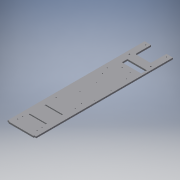
# Autodesk Inventor part: Control Board
Saved by Autodesk Inventor 2016 (Build 200138000, 138)
## iProperties
Created: 2017-09-15
Part Number: Control Board
Material: Generic
Document SubType Name: Modeling
Designer: Student
Density: 1 g/cm^3
Appearance: Default
Author: Student
Autodesk Inventor part; units mm, degrees
ref_plane "YZ Plane" through (0, 0, 0) normal (1, 0, 0) x (0, 1, 0)
ref_plane "XZ Plane" through (0, 0, 0) normal (0, 1, 0) x (-1, 0, 0)
ref_plane "XY Plane" through (0, 0, 0) normal (0, 0, 1) x (1, 0, 0)
sketch "Sketch1" plane through (0, 0, 0) normal (0, 1, 0) x (-1, 0, 0)
  line L0 (47.9603, 101.1149) -> (-52.1157, 101.1149)
  line L1 (-52.1157, 101.1149) -> (-52.1157, -254.4851)
  line L2 (-52.1157, -254.4851) -> (47.9603, -254.4851)
  line L3 (47.9603, -254.4851) -> (47.9603, 101.1149)
  point P0 (0, 0)
  dimension "d0" = 100.076
  dimension "d1" = 355.6
  constraints: 8 end point, 2 parallel, 1 horizontal, 1 perpendicular
  measures "d0" distance of L0.start L0.end
  measures "d1" distance of L2.end L0.start
extrude "Extrusion1" add sketch "Sketch1" along normal blind 5.4102
sketch "Sketch5" plane through (0, 5.4102, 0) normal (0, 1, 0) x (1, 0, 0)
  circle A0 centre (-34.7523, 244.8585) radius 1.5
  circle A1 centre (38.9077, 244.8585) radius 1.5
  line L0 (-34.7355, 243.3586) -> (38.8909, 243.3586)
  line L1 (52.1157, 254.4851) -> (-47.9603, 254.4851) projected
  point P0 (0, 0)
  point P1 (2.0777, 243.3586)
  point P2 (2.0777, 254.4851)
  dimension "d8" = 3
  dimension "d9" = 3
  dimension "d10" = 73.66
  dimension "d11" = 9.6266
  constraints: 2 end point, 2 midpoint, 1 horizontal, 1 vertical alignment, 6 other
  measures "d10" distance of point (38.908, 244.859) point (-34.752, 244.859)
  measures "d11" distance from line of L1 point (38.908, 244.859)
extrude "Extrusion3" cut sketch "Sketch5" against normal blind 25.4
sketch "Sketch6" plane through (0, 5.4102, 0) normal (0, 1, 0) x (1, 0, 0)
  line L0 (-47.9603, -101.1149) -> (52.1157, -101.1149) projected
  line L1 (-47.9603, -101.1149) -> (-41.6103, -101.1149)
  line L2 (-41.6103, -101.1149) -> (-41.6103, -98.3209)
  line L3 (-41.6103, -98.3209) -> (-47.9603, -98.3209)
  line L4 (-47.9603, -98.3209) -> (-47.9603, -101.1149)
  line L5 (52.1157, -101.1149) -> (45.7657, -101.1149)
  line L6 (45.7657, -101.1149) -> (45.7657, -98.3209)
  line L7 (45.7657, -98.3209) -> (52.1157, -98.3209)
  line L8 (52.1157, -98.3209) -> (52.1157, -101.1149)
  point P0 (0, 0)
  dimension "d14" = 2.794
  dimension "d15" = 6.35
  dimension "d16" = 6.35
  constraints: 16 end point, 4 parallel, 2 horizontal, 2 perpendicular, 1 point on line
  measures "d14" distance of L1.end L2.end
  measures "d15" distance of L2.end L3.end
  measures "d16" distance of L6.end L7.end
extrude "Extrusion4" cut sketch "Sketch6" against normal blind 25.4
sketch "Sketch7" plane through (45.7657, 5.4102, 98.3209) normal (0, 0, 1) x (1, 0, 0)
  circle A0 centre (3.175, -2.7051) radius 1.5
  line L0 (0, 0) -> (6.35, 0) projected
  line L1 (6.35, 0) -> (6.35, -5.4102) projected
  circle A1 centre (-90.551, -2.7051) radius 1.5
  line L2 (-93.726, 0) -> (-87.376, 0) projected
  line L3 (-93.726, -5.4102) -> (-93.726, 0) projected
  point P0 (-45.7657, -5.4102)
  point P1 (3.175, 0)
  point P2 (6.35, -2.7051)
  point P3 (-90.551, 0)
  point P4 (-93.726, -2.7051)
  dimension "d19" = 3
  dimension "d20" = 3
  constraints: 4 midpoint, 2 centre point, 2 horizontal alignment, 2 vertical alignment
  measures "d19" diameter of A0
  measures "d20" diameter of A1
extrude "Extrusion5" cut sketch "Sketch7" against normal blind 254
sketch "Sketch8" plane through (-41.6103, 0, 101.1149) normal (0, 0, 1) x (1, 0, 0)
  line L0 (0, 5.4102) -> (87.376, 5.4102) projected
  line L1 (0, 0) -> (87.376, 0) projected
  line L2 (0, 5.4102) -> (87.376, 5.4102)
  line L3 (87.376, 5.4102) -> (87.376, 0)
  line L4 (87.376, 0) -> (0, 0)
  line L5 (0, 0) -> (0, 5.4102)
  point P0 (41.6103, 0)
  constraints: 8 end point, 2 parallel, 1 horizontal, 1 perpendicular
extrude "Extrusion6" add sketch "Sketch8" along normal blind 54.5338
sketch "Sketch9" plane through (-47.9603, 5.4102, 98.3209) normal (0, 0, 1) x (1, 0, 0)
  line L0 (6.35, 0) -> (6.35, -5.4102) projected
  line L1 (0, 0) -> (6.35, 0)
  line L2 (6.35, 0) -> (6.35, -5.4102)
  line L3 (6.35, -5.4102) -> (0, -5.4102)
  line L4 (0, -5.4102) -> (0, 0)
  line L5 (100.076, 0) -> (100.076, -5.4102) projected
  line L6 (100.076, -5.4102) -> (93.726, -5.4102) projected
  line L7 (100.076, 0) -> (93.726, 0)
  line L8 (93.726, 0) -> (93.726, -5.4102)
  line L9 (93.726, -5.4102) -> (100.076, -5.4102)
  line L10 (100.076, -5.4102) -> (100.076, 0)
  circle A0 centre (96.901, -2.7051) radius 1.5
  circle A1 centre (3.175, -2.7051) radius 1.5
  point P0 (47.9603, -5.4102)
  constraints: 16 end point, 4 parallel, 2 centre point, 2 horizontal, 2 perpendicular
extrude "Extrusion7" add sketch "Sketch9" along normal blind 54.5338
sketch "Sketch10" plane through (0, 5.4102, 0) normal (0, 1, 0) x (1, 0, 0)
  line L0 (-37.6261, -131.8997) -> (38.5739, -131.8997) construction
  line L1 (-37.6261, -106.4997) -> (38.5739, -106.4997) construction
  line L2 (-47.9603, 254.4851) -> (-47.9603, -152.8547) construction
  line L3 (52.1157, -152.8547) -> (52.1157, 254.4851) construction
  line L4 (45.7657, -155.6487) -> (-41.6103, -155.6487) construction
  line L5 (-37.6261, -114.1197) -> (-12.2261, -114.1197) construction
  line L6 (-12.2261, -114.1197) -> (-12.2261, -124.2797) construction
  line L7 (-12.2261, -124.2797) -> (-37.6261, -124.2797) construction
  line L8 (-37.6261, -131.8997) -> (-37.6261, -124.2797) construction
  line L9 (-37.6261, -114.1197) -> (-37.6261, -106.4997) construction
  line L10 (38.5739, -114.1197) -> (13.1739, -114.1197) construction
  line L11 (13.1739, -114.1197) -> (13.1739, -124.2797) construction
  line L12 (13.1739, -124.2797) -> (38.5739, -124.2797) construction
  line L13 (38.5739, -131.8997) -> (38.5739, -124.2797) construction
  line L14 (38.5739, -114.1197) -> (38.5739, -106.4997) construction
  circle A0 centre (34.7639, -110.3097) radius 1.5
  circle A1 centre (34.7639, -128.0897) radius 1.5
  circle A2 centre (-33.816, -127.9782) radius 1.5
  circle A3 centre (-33.816, -110.1982) radius 1.5
  point P0 (0, 0)
  point P1 (38.5739, -110.3097)
  dimension "d27" = 76.2
  dimension "d28" = 25.4
  dimension "d31" = 23.749
  dimension "d32" = 7.62
  dimension "d33" = 7.62
  dimension "d34" = 25.4
  dimension "d35" = 25.4
  dimension "d36" = 68.58
  dimension "d37" = 17.78
  dimension "d38" = 17.78
  dimension "d39" = 68.58
  dimension "d40" = 3
  dimension "d41" = 3
  dimension "d42" = 3
  dimension "d43" = 3
  dimension "d44" = 3.81
  dimension "d45" = 25.4
  dimension "d46" = 25.4
  dimension "d47" = 7.62
  dimension "d48" = 7.62
  dimension "d49" = 7.62
  dimension "d50" = 7.62
  dimension "d51" = 76.2
  dimension "d52" = 25.4
  dimension "d53" = 25.4
  dimension "d54" = 17.78
  constraints: 24 end point, 12 perpendicular, 4 centre point, 2 horizontal, 2 vertical, 2 vertical alignment, 1 horizontal alignment, 1 midpoint
  measures "d27" distance of L1.start L1.end
  measures "d28" distance of L0.start L1.start
  measures "d31" distance between parallel lines of L4 L0
  measures "d32" distance between parallel lines of L1 L5
  measures "d33" distance between parallel lines of L7 L0
  measures "d34" distance of L5.start L5.end
  measures "d35" distance of L10.start L10.end
  measures "d36" distance of A3.centre A0.centre
  measures "d37" distance of A1.centre A0.centre
  measures "d38" distance of A3.centre A2.centre
  measures "d39" distance of A1.centre A2.centre
  measures "d40" diameter of A3
  measures "d41" diameter of A2
  measures "d42" diameter of A0
  measures "d43" diameter of A1
  measures "d44" distance from line of L14 A0.centre
  measures "d45" distance of L11.end L12.end
  measures "d46" distance of L6.end L7.end
  measures "d47" distance of L5.start L1.start
  measures "d48" distance of L10.start L1.end
  measures "d49" distance of L0.end L12.end
  measures "d50" distance of L0.start L7.end
  measures "d51" distance of L0.start L0.end
  measures "d52" distance between parallel lines of L11 L6
  measures "d53" distance between parallel lines of L0 L1
  measures "d54" distance of A2.centre A3.centre
extrude "Extrusion8" cut sketch "Sketch10" against normal blind 54.5338
sketch "Sketch11" plane through (0, 5.4102, 0) normal (0, 1, 0) x (1, 0, 0)
  line L0 (-41.6103, -155.6487) -> (45.7657, -155.6487) construction
  line L1 (43.9115, -155.6487) -> (43.9115, -13.9421) construction
  line L2 (43.9115, -13.9421) -> (52.1157, -13.9421) construction
  line L3 (52.1157, -152.8547) -> (52.1157, 254.4851) construction
  circle A0 centre (43.9115, -13.9421) radius 1.0922
  circle A1 centre (-7.8029, -13.9421) radius 1.0922
  circle A2 centre (43.9115, 43.9953) radius 1.0928
  circle A3 centre (-7.8029, 43.9953) radius 1.0922
  point P0 (0, 0)
  dimension "d57" = 141.7066
  dimension "d58" = 8.2042
  dimension "d59" = 2.1844
  dimension "d60" = 2.1844
  dimension "d62" = 51.7144
  dimension "d63" = 57.9374
  dimension "d64" = 57.9374
  constraints: 4 centre point, 4 end point, 2 point on line, 1 coincident, 1 perpendicular, 1 vertical
  measures "d57" distance of L1.start L1.end
  measures "d58" distance of L1.end L2.end
  measures "d59" diameter of A0
  measures "d60" diameter of A1
  measures "d62" distance of L1.end A1.centre
  measures "d63" distance of L1.end A2.centre
  measures "d64" distance of A3.centre A1.centre
extrude "Extrusion9" cut sketch "Sketch11" against normal blind 54.5338
sketch "Sketch12" plane through (0, 5.4102, 0) normal (0, 1, 0) x (1, 0, 0)
  circle A0 centre (43.4543, 73.8403) radius 1.5367
  line L0 (52.1157, -152.8547) -> (52.1157, 254.4851) projected
  line L1 (52.1157, -152.8547) -> (45.7657, -152.8547) projected
  line L2 (46.0959, 58.6257) -> (46.0959, 133.7589) construction
  line L3 (46.0959, 58.6257) -> (-7.3203, 58.6257) construction
  line L4 (46.0959, 133.7589) -> (44.0639, 133.7589) construction
  line L5 (44.0639, 133.7589) -> (44.0639, 136.7053) construction
  line L6 (44.0639, 136.7053) -> (6.6751, 136.7053) construction
  line L7 (6.6751, 136.7053) -> (6.6751, 133.7589) construction
  line L8 (6.6751, 133.7589) -> (-7.2949, 133.7589) construction
  line L9 (-7.3203, 58.6257) -> (-7.2949, 133.7589) construction
  circle A1 centre (38.5521, 134.0637) radius 1.5367
  circle A2 centre (10.6629, 134.0637) radius 1.5367
  point P0 (0, 0)
  dimension "d67" = 3.0734
  dimension "d68" = 8.6614
  dimension "d69" = 226.695
  dimension "d89" = 15.2146
  dimension "d90" = 2.6416
  dimension "d91" = 75.1332
  dimension "d92" = 53.4162
  dimension "d93" = 2.032
  dimension "d94" = 2.9464
  dimension "d95" = 37.3888
  dimension "d96" = 13.97
  dimension "d97" = 75.1332
  dimension "d98" = 3.0734
  dimension "d99" = 2.6416
  dimension "d100" = 3.0734
  dimension "d101" = 2.6416
  dimension "d102" = 27.8892
  dimension "d103" = 7.5438
  dimension "d104" = 60.4226
  constraints: 16 end point, 3 centre point, 3 horizontal, 3 vertical, 1 perpendicular
  measures "d67" diameter of A0
  measures "d68" distance from line of L0 A0.centre
  measures "d69" distance from line of A0.centre L1
  measures "d89" distance from line of L3 A0.centre
  measures "d90" distance from line of L2 A0.centre
  measures "d91" distance of L2.start L2.end
  measures "d92" distance of L2.start L3.end
  measures "d93" distance of L2.end L4.end
  measures "d94" distance of L4.end L5.end
  measures "d95" distance of L5.end L6.end
  measures "d96" distance of L7.end L8.end
  measures "d97" distance of L3.end L8.end
  measures "d98" diameter of A1
  measures "d99" distance from line of L6 A1.centre
  measures "d100" diameter of A2
  measures "d101" distance from line of L6 A2.centre
  measures "d102" distance of A1.centre A2.centre
  measures "d103" distance from line of L2 A1.centre
  measures "d104" distance of A1.centre A0.centre
extrude "Extrusion10" cut sketch "Sketch12" against normal blind 25.4
sketch "Sketch13" plane through (0, 5.4102, 0) normal (0, 1, 0) x (1, 0, 0)
  line L0 (44.9886, 149.6605) -> (-23.5191, 149.6605)
  line L1 (-23.5191, 149.6605) -> (-23.5191, 169.3907)
  line L2 (-23.5191, 169.3907) -> (44.9886, 169.3907)
  line L3 (44.9886, 169.3907) -> (44.9886, 149.6605)
  point P0 (0, 0)
  constraints: 8 end point, 2 parallel, 1 horizontal, 1 perpendicular
extrude "Extrusion11" cut sketch "Sketch13" against normal blind 25.4
sketch "Sketch14" plane through (0, 5.4102, 0) normal (0, 1, 0) x (1, 0, 0)
  line L0 (-39.2837, 182.0907) -> (45.1561, 182.0907) construction
  line L1 (45.1561, 182.0907) -> (45.1561, 192.9873) construction
  line L2 (45.1561, 192.9873) -> (-39.2837, 192.9873) construction
  line L3 (-39.2837, 192.9873) -> (-39.2837, 182.0907) construction
  line L4 (-23.5191, 169.3907) -> (44.9886, 169.3907) construction
  circle A0 centre (40.7951, 187.539) radius 2.2274
  circle A1 centre (-34.9227, 187.539) radius 2.2274
  line L5 (-47.9603, 254.4851) -> (-47.9603, -152.8547) construction
  line L6 (52.1157, -152.8547) -> (52.1157, 254.4851) construction
  point P0 (0, 0)
  dimension "d107" = 84.4398
  dimension "d108" = 10.8966
  dimension "d109" = 12.7
  dimension "d110" = 2.1336
  dimension "d111" = 2.1336
  dimension "d114" = 6.9596
  constraints: 8 end point, 3 perpendicular, 2 centre point, 1 horizontal
  measures "d107" distance of L1.end L2.end
  measures "d108" distance of L2.end L0.start
  measures "d109" distance between parallel lines of L4 L0
  measures "d110" distance edge to line of A0 L1
  measures "d111" distance edge to line of A1 L3
  measures "d114" distance between parallel lines of L6 L1
extrude "Extrusion12" cut sketch "Sketch14" against normal blind 25.4
sketch "Sketch15" plane through (0, 5.4102, 0) normal (0, 1, 0) x (1, 0, 0)
  circle A0 centre (30.5257, -47.4955) radius 1.5
  line L0 (-47.9603, 254.4851) -> (-47.9603, -152.8547) projected
  line L1 (-41.6103, -152.8547) -> (-47.9603, -152.8547) projected
  line L2 (52.1157, -152.8547) -> (52.1157, 254.4851) projected
  circle A1 centre (-24.0589, 81.4603) radius 1.5
  point P0 (0, 0)
  dimension "d117" = 3
  dimension "d119" = 105.3592
  dimension "d120" = 21.59
  dimension "d121" = 3
  dimension "d122" = 23.9014
  dimension "d123" = 234.315
  constraints: 2 centre point
  measures "d117" diameter of A0
  measures "d119" distance from line of L1 A0.centre
  measures "d120" distance from line of L2 A0.centre
  measures "d121" diameter of A1
  measures "d122" distance from line of L0 A1.centre
  measures "d123" distance from line of L1 A1.centre
extrude "Extrusion13" cut sketch "Sketch15" against normal blind 25.4
sketch "Sketch16" plane through (0, 0, 0) normal (0, -1, 0) x (1, 0, 0)
  line L0 (38.0609, 76.6965) -> (-35.2689, 76.6965)
  line L1 (-35.2689, 76.6965) -> (-35.2689, -110.1035)
  line L2 (-35.2689, -110.1035) -> (38.0609, -110.1035)
  line L3 (38.0609, -110.1035) -> (38.0609, 76.6965)
  circle A0 centre (35.0609, 73.6965) radius 1.5
  circle A1 centre (-32.2689, 73.6965) radius 1.5
  circle A2 centre (-32.2689, -107.1035) radius 1.5
  circle A3 centre (35.0609, -107.1035) radius 1.5
  point P0 (0, 0)
  dimension "d128" = 186.8
  dimension "d129" = 73.3298
  dimension "d130" = 3
  dimension "d131" = 3
  dimension "d132" = 3
  dimension "d133" = 3
  dimension "d134" = 3
  dimension "d135" = 3
  dimension "d136" = 3
  dimension "d137" = 3
  dimension "d138" = 3
  dimension "d139" = 3
  dimension "d140" = 3
  dimension "d141" = 3
  constraints: 8 end point, 4 centre point, 2 parallel, 1 horizontal, 1 perpendicular
  measures "d128" distance of L2.end L0.start
  measures "d129" distance of L1.end L2.end
  measures "d130" diameter of A0
  measures "d131" distance from line of L3 A0.centre
  measures "d132" distance from line of L0 A0.centre
  measures "d133" distance from line of L1 A1.centre
  measures "d134" distance from line of L0 A1.centre
  measures "d135" diameter of A1
  measures "d136" diameter of A2
  measures "d137" distance from line of L2 A2.centre
  measures "d138" distance from line of L1 A2.centre
  measures "d139" diameter of A3
  measures "d140" distance from line of L2 A3.centre
  measures "d141" distance from line of L3 A3.centre
extrude "Extrusion14" cut sketch "Sketch16" against normal blind 25.4 contours A0 | A1 | A2 | A3
sketch "Sketch17" plane through (-41.6103, 0, 155.6487) normal (0, 0, 1) x (1, 0, 0)
  line L0 (0, 5.4102) -> (0, 0) projected
  line L1 (0, 0) -> (87.376, 0) projected
  line L2 (0, 5.4102) -> (87.376, 5.4102)
  line L3 (87.376, 5.4102) -> (87.376, 0)
  line L4 (87.376, 0) -> (0, 0)
  line L5 (0, 0) -> (0, 5.4102)
  point P0 (41.6103, 0)
  constraints: 8 end point, 2 parallel, 1 horizontal, 1 perpendicular
sketch "Sketch18" plane through (-47.9603, 5.4102, 152.8547) normal (0, 0, 1) x (1, 0, 0)
  line L0 (100.076, 0) -> (0, 0) projected
  line L1 (0, -5.4102) -> (6.35, -5.4102) projected
  line L2 (0, 0) -> (6.35, 0)
  line L3 (6.35, 0) -> (6.35, -5.4102)
  line L4 (6.35, -5.4102) -> (0, -5.4102)
  line L5 (0, -5.4102) -> (0, 0)
  circle A0 centre (3.175, -2.7051) radius 1.5
  line L6 (93.726, -5.4102) -> (93.726, 0) projected
  line L7 (100.076, -5.4102) -> (100.076, 0) projected
  line L8 (93.726, 0) -> (100.076, 0)
  line L9 (100.076, 0) -> (100.076, -5.4102)
  line L10 (100.076, -5.4102) -> (93.726, -5.4102)
  line L11 (93.726, -5.4102) -> (93.726, 0)
  circle A1 centre (96.901, -2.7051) radius 1.5
  point P0 (47.9603, -5.4102)
  constraints: 16 end point, 4 parallel, 2 centre point, 2 horizontal, 2 perpendicular
extrude "Extrusion15" add sketch "Sketch17" along normal blind 76.2
extrude "Extrusion16" add sketch "Sketch18" along normal blind 76.2
sketch "Sketch19" plane through (0, 5.4102, 0) normal (0, 1, 0) x (1, 0, 0)
  circle A0 centre (-33.816, -127.9782) radius 1.5 projected
  circle A1 centre (-33.816, -127.9782) radius 1.5
  circle A2 centre (34.7639, -128.0897) radius 1.5 projected
  circle A3 centre (34.7639, -128.0897) radius 1.5
  circle A4 centre (-33.816, -208.3096) radius 1.5
  circle A5 centre (-33.816, -190.5296) radius 1.5
  circle A6 centre (34.7639, -190.5296) radius 1.5
  circle A7 centre (34.7639, -208.3096) radius 1.5
  point P0 (0, 0)
  dimension "d148" = 3
  dimension "d149" = 3
  dimension "d150" = 3
  dimension "d151" = 3
  dimension "d152" = 17.78
  dimension "d153" = 17.78
  dimension "d154" = 68.5799
  dimension "d155" = 68.5799
  dimension "d156" = 68.5799
  constraints: 6 centre point, 2 coincident
  measures "d148" diameter of A7
  measures "d149" diameter of A6
  measures "d150" diameter of A5
  measures "d151" diameter of A4
  measures "d152" distance of A5.centre A4.centre
  measures "d153" distance of A6.centre A7.centre
  measures "d154" distance of A3.centre A1.centre
  measures "d155" distance of A6.centre A5.centre
  measures "d156" distance of A7.centre A4.centre
extrude "Extrusion17" cut sketch "Sketch19" against normal blind 25.4 contours A4 | A5 | A6 | A7
sketch "Sketch20" plane through (0, 5.4102, 0) normal (0, 1, 0) x (1, 0, 0)
  circle A0 centre (-33.816, -127.9782) radius 1.5 projected
  circle A1 centre (-33.816, -127.9782) radius 1.5
  circle A2 centre (-33.816, -110.1982) radius 1.5 projected
  circle A3 centre (-33.816, -110.1982) radius 1.5
  circle A4 centre (34.7639, -110.3097) radius 1.5 projected
  circle A5 centre (34.7639, -110.3097) radius 1.5
  circle A6 centre (34.7639, -128.0897) radius 1.5 projected
  circle A7 centre (34.7639, -128.0897) radius 1.5
  point P0 (0, 0)
  constraints: 4 centre point, 4 coincident
extrude "Extrusion18" add sketch "Sketch20" against normal blind 5.4102
sketch "Sketch21" plane through (0, 5.4102, 0) normal (0, 1, 0) x (1, 0, 0)
  circle A0 centre (-6.6492, 134.0637) radius 1.5
  circle A1 centre (21.24, 134.0637) radius 1.5
  circle A2 centre (10.6629, 134.0637) radius 1.5367 projected
  circle A3 centre (10.6629, 134.0637) radius 1.5367
  circle A4 centre (38.5521, 134.0637) radius 1.5367 projected
  circle A5 centre (38.5521, 134.0637) radius 1.5367
  point P0 (0, 0)
  dimension "d161" = 3
  dimension "d162" = 3
  dimension "d163" = 27.8892
  dimension "d164" = 27.8892
  constraints: 4 centre point, 2 coincident, 1 horizontal alignment
  measures "d161" diameter of A1
  measures "d162" diameter of A0
  measures "d163" distance of A5.centre A3.centre
  measures "d164" distance of A0.centre A1.centre
extrude "Extrusion19" cut sketch "Sketch21" against normal blind 5.4102 contours A0 | A1
sketch "Sketch22" plane through (0, 5.4102, 0) normal (0, 1, 0) x (1, 0, 0)
  line L0 (42.3287, 131.8326) -> (35.2249, 131.8326)
  line L1 (35.2249, 131.8326) -> (35.2249, 136.3465)
  line L2 (35.2249, 136.3465) -> (42.3287, 136.3465)
  line L3 (42.3287, 136.3465) -> (42.3287, 131.8326)
  line L4 (13.9876, 131.1666) -> (7.1058, 131.1666)
  line L5 (7.1058, 131.1666) -> (7.1058, 137.7525)
  line L6 (7.1058, 137.7525) -> (13.9876, 137.7525)
  line L7 (13.9876, 137.7525) -> (13.9876, 131.1666)
  line L8 (47.4407, -229.0547) -> (47.4407, 155.6791) projected
  line L9 (36.9122, 68.1776) -> (47.4407, 68.1776)
  line L10 (47.4407, 68.1776) -> (47.4407, 78.0252)
  line L11 (47.4407, 78.0252) -> (36.9122, 78.0252)
  line L12 (36.9122, 78.0252) -> (36.9122, 68.1776)
  point P0 (0, 0)
  constraints: 24 end point, 6 parallel, 3 horizontal, 3 perpendicular, 1 point on line
extrude "Extrusion20" add sketch "Sketch22" against normal blind 5.4102
sketch "Sketch23" plane through (0, 0, 0) normal (0, -1, 0) x (1, 0, 0)
  line L0 (-28.8727, 170.2662) -> (31.8492, 170.2662)
  line L1 (31.8492, 170.2662) -> (31.8492, 174.0762)
  line L2 (31.8492, 174.0762) -> (-28.8727, 174.0762)
  line L3 (-28.8727, 174.0762) -> (-28.8727, 170.2662)
  line L4 (-28.8727, 117.8628) -> (31.8492, 117.8628)
  line L5 (31.8492, 117.8628) -> (31.8492, 114.0528)
  line L6 (31.8492, 114.0528) -> (-28.8727, 114.0528)
  line L7 (-28.8727, 114.0528) -> (-28.8727, 117.8628)
  point P0 (0, 0)
  dimension "d169" = 3.81
  dimension "d170" = 3.81
  constraints: 16 end point, 4 parallel, 2 horizontal, 2 perpendicular
  measures "d169" distance of L2.end L0.start
  measures "d170" distance of L6.end L4.start
extrude "Extrusion21" cut sketch "Sketch23" against normal blind 5.4102
sketch "Sketch24" plane through (0, 5.4102, 0) normal (0, 1, 0) x (1, 0, 0)
  line L0 (52.1157, 254.4851) -> (-47.9603, 254.4851) projected
  line L1 (-25.1257, 254.4851) -> (29.2811, 254.4851)
  line L2 (29.2811, 254.4851) -> (29.2811, 198.5828)
  line L3 (29.2811, 198.5828) -> (-25.1257, 198.5828)
  line L4 (-25.1257, 198.5828) -> (-25.1257, 254.4851)
  line L5 (-47.9603, 254.4851) -> (-47.9603, -229.0547) projected
  line L6 (52.1157, -229.0547) -> (52.1157, 254.4851) projected
  point P0 (0, 0)
  dimension "d173" = 22.8346
  dimension "d174" = 22.8346
  constraints: 8 end point, 2 parallel, 1 horizontal, 1 perpendicular, 1 point on line
  measures "d173" distance between parallel lines of L5 L4
  measures "d174" distance between parallel lines of L6 L2
extrude "Extrusion22" cut sketch "Sketch24" against normal blind 5.4102
fillet "Fillet1" radius 3.175 2 edges at (29.2811, 2.7051, -198.5828) (-25.1257, 2.7051, -198.5828)
equation "\"d9\" = d8"
equation "\"d20\" = d19"
equation "\"d60\" = d59"
equation "\"d111\" = d110"
equation "\"d121\" = d117"
equation "\"d164\" = d163"
equation "\"d170\" = d169"
body "Solid1"
